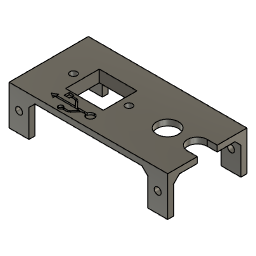
Rear USB Port (Autodesk Fusion 360 design; units mm, degrees)
Autodesk Fusion 360 part; units mm, degrees
note: some values were not read from the file. Set by a fixed rule: which sketch regions a step uses.
sketch "Sketch1" plane through (0, 0, 0) normal (0, 0, 1) x (1, 0, 0)
  line L0 (40, -20) -> (-40, -20)
  line L1 (-40, -20) -> (-40, 20)
  line L2 (-40, 20) -> (40, 20)
  line L3 (40, 20) -> (40, -20)
  line L4 (-20, 5.5) -> (-7, 5.5)
  line L5 (-7, 5.5) -> (-7, -5.5)
  line L6 (-7, -5.5) -> (-20, -5.5)
  line L7 (-20, -5.5) -> (-20, 5.5)
  circle A0 centre (-27.5, 0) radius 1.75
  circle A1 centre (0.5, 0) radius 1.75
  line L8 (-40, -20) -> (-30, -20)
  line L9 (-30, -20) -> (-30, -17)
  line L10 (-30, -17) -> (-40, -17)
  line L11 (-40, -17) -> (-40, -20)
  line L12 (-40, 20) -> (-30, 20)
  line L13 (-30, 20) -> (-30, 17)
  line L14 (-30, 17) -> (-40, 17)
  line L15 (-40, 17) -> (-40, 20)
  line L16 (40, 20) -> (30, 20)
  line L17 (30, 20) -> (30, 17)
  line L18 (30, 17) -> (40, 17)
  line L19 (40, 17) -> (40, 20)
  line L20 (40, -20) -> (30, -20)
  line L21 (30, -20) -> (30, -17)
  line L22 (30, -17) -> (40, -17)
  line L23 (40, -17) -> (40, -20)
  circle A2 centre (20, 0) radius 5.5
  circle A3 centre (35, 0) radius 5
  line L24 (35, 5) -> (35.7366, 5)
  line L25 (35.7366, 5) -> (40, 5)
  line L26 (34.9626, -4.9999) -> (35.7366, -5.0056)
  line L27 (35.7366, -5.0056) -> (40, -5.0056)
  dimension "d1" = 80
  dimension "d2" = 40
  dimension "d3" = 13
  dimension "d4" = 11
  dimension "d5" = 5.5
  dimension "d7" = 3.5
  dimension "d8" = 3.5
  dimension "d9" = 7.5
  dimension "d10" = 7.5
  dimension "d11" = 5.5
  dimension "d12" = 5.5
  dimension "d13" = 10
  dimension "d14" = 3
  dimension "d15" = 3
  dimension "d16" = 10
  dimension "d17" = 3
  dimension "d18" = 10
  dimension "d19" = 10
  dimension "d20" = 3
  dimension "d36" = 14.5
  dimension "d38" = 20
  dimension "d39" = 40
  dimension "d40" = 11
  dimension "d42" = 20
  dimension "d43" = 10
  dimension "d44" = 5
  dimension "d45" = 15
  constraint perpendicular L0 L1
  constraint parallel L0 L2
  constraint parallel L1 L3
  constraint horizontal L0
  constraint horizontal L4
  constraint vertical L5
  constraint horizontal L6
  constraint vertical L7
  constraint horizontal L8
  constraint vertical L9
  constraint horizontal L10
  constraint vertical L11
  constraint horizontal L12
  constraint vertical L13
  constraint horizontal L14
  constraint vertical L15
  constraint horizontal L16
  constraint vertical L17
  constraint horizontal L18
  constraint vertical L19
  constraint horizontal L20
  constraint vertical L21
  constraint horizontal L22
  constraint vertical L23
  constraint coincident A3 L24.start
  constraint tangent A3 L24
  constraint perpendicular L3 L24
  constraint coincident L3 L25.end
  constraint perpendicular L3 L25
  constraint coincident A3 L26.start
  constraint tangent A3 L26
  constraint coincident L3 L27.end
  constraint perpendicular L3 L27
  measures "d1" distance of L1.end L2.end
  measures "d2" distance of L0.end L1.end
  measures "d3" distance of L4.start L4.end
  measures "d4" distance of L4.start L6.end
  measures "d5" distance of origin L4
  measures "d7" diameter of A0
  measures "d8" diameter of A1
  measures "d9" distance of L5 A1.centre
  measures "d10" distance of L7 A0.centre
  measures "d11" distance of L4 A1.centre
  measures "d12" distance of L4 A0.centre
  measures "d13" distance of L0.end L8.end
  measures "d14" distance of L0.end L10.end
  measures "d15" distance of L1.end L14.end
  measures "d16" distance of L1.end L12.end
  measures "d17" distance of L2.end L18.end
  measures "d18" distance of L2.end L16.end
  measures "d19" distance of L0.start L20.end
  measures "d20" distance of L0.start L22.end
  measures "d36" distance of L2 L4
  measures "d38" distance of L1 L7
  measures "d39" distance of L3 origin
  measures "d40" diameter of A2
  measures "d42" distance of L2 A2.centre
  measures "d43" diameter of A3
  measures "d44" distance of L3 A3.centre
  measures "d45" distance of A2.centre A3.centre
extrude "Extrude1" add sketch "Sketch1" along normal blind 3 contours L0 L3 L20 L21 L22 L23 | L0 L1 L2 L3 L9 L10 L13 L14 L17 L18 L21 L22 A3 L24 L25 L26 L27 | L0 L1 L8 L9 L10 L11 | L1 L2 L12 L13 L14 L15 | L2 L3 L16 L17 L18 L19
extrude "Extrude2" add sketch "Sketch1" against normal blind 17 contours L0 L3 L20 L21 L22 L23 | L0 L1 L8 L9 L10 L11 | L1 L2 L12 L13 L14 L15 | L2 L3 L16 L17 L18 L19
sketch "Sketch2" plane through (0, -20, 0) normal (0, -1, 0) x (1, 0, 0)
  line L0 (-30, 0) -> (30, 0)
  line L1 (30, 0) -> (30, -17)
  line L2 (30, -17) -> (40, -17)
  line L3 (40, -17) -> (40, 3)
  line L4 (40, 3) -> (-40, 3)
  line L5 (-40, 3) -> (-40, -17)
  line L6 (-40, -17) -> (-30, -17)
  line L7 (-30, -17) -> (-30, 0)
  circle A0 centre (35, -7) radius 1.75
  circle A1 centre (-35, -7) radius 1.75
  dimension "d25" = 3.5
  dimension "d26" = 10
  dimension "d27" = 5
  dimension "d28" = 3.5
  dimension "d29" = 5
  dimension "d30" = 10
  measures "d25" diameter of A0
  measures "d26" distance of L4 A0.centre
  measures "d27" distance of L3 A0.centre
  measures "d28" diameter of A1
  measures "d29" distance of L5 A1.centre
  measures "d30" distance of L4 A1.centre
extrude "Extrude3" cut sketch "Sketch2" against normal up to surface (40 mm away) contours A0 | A1
chamfer "Chamfer1" distance 3 angle 45 4 edges at (-7, 0, 3) (-13.5, 5.5, 3) (-20, 0, 3) (-13.5, -5.5, 3)
sketch "Sketch3" plane through (0, 0, 3) normal (0, 0, 1) x (-1, 0, 0)
  line L0 (-40, -5) -> (-40, -20)
  line L1 (-40, -20) -> (40, -20)
  line L2 (40, -20) -> (40, 20)
  circle A0 centre (27.5, 0) radius 1.75
  circle A1 centre (-0.5, 0) radius 1.75
  line L3 (23, 8.5) -> (23, -8.5)
  line L4 (23, -8.5) -> (4, -8.5)
  line L5 (4, -8.5) -> (4, 8.5)
  line L6 (4, 8.5) -> (23, 8.5)
  line L7 (24.6533, 14.1697) -> (22.2252, 15.5719)
  line L8 (22.2252, 15.5719) -> (22.2252, 14.5716)
  line L9 (22.2252, 14.5716) -> (9.8144, 14.5716)
  line L10 (9.8144, 14.5716) -> (12.2309, 17.1247)
  spline S0 degree 3 poles (12.2309, 17.1247) (12.4366, 17.2895) (12.7057, 17.4052) (12.9824, 17.4116) knots 0 0 0 0 1 1 1 1
  spline S1 degree 3 poles (12.9824, 17.4116) (14.1022, 17.4116) (14.7671, 17.4119) (15.0119, 17.4123) knots 0 0 0 0 1 1 1 1
  spline S2 degree 3 poles (15.0119, 17.4123) (15.1778, 16.9396) (15.6235, 16.5985) (16.1533, 16.5985) knots 0 0 0 0 1 1 1 1
  spline S3 degree 3 poles (16.1533, 16.5985) (16.8235, 16.5985) (17.3675, 17.1423) (17.3675, 17.8128) knots 0 0 0 0 1 1 1 1
  spline S4 degree 3 poles (17.3675, 17.8128) (17.3675, 18.4836) (16.8236, 19.0273) (16.1533, 19.0273) knots 0 0 0 0 1 1 1 1
  spline S5 degree 3 poles (16.1533, 19.0273) (15.6235, 19.0273) (15.1778, 18.6863) (15.0119, 18.214) knots 0 0 0 0 1 1 1 1
  line L11 (15.0119, 18.214) -> (13.0062, 18.2143)
  spline S6 degree 3 poles (13.0062, 18.2143) (12.4626, 18.2143) (11.893, 17.9161) (11.5305, 17.5665) knots 0 0 0 0 1 1 1 1
  spline S7 degree 3 poles (11.5305, 17.5665) (11.5404, 17.5768) (11.5507, 17.5879) (11.5299, 17.5663) knots 0 0 0 0 1 1 1 1
  spline S8 degree 2 poles (11.5299, 17.5663) (11.5222, 17.5576) (8.9661, 14.8578) knots 0 0 0 1 1 1
  spline S9 degree 3 poles (8.9661, 14.8578) (8.7609, 14.6932) (8.4919, 14.5783) (8.2153, 14.5717) knots 0 0 0 0 1 1 1 1
  line L12 (8.2153, 14.5717) -> (6.8114, 14.5717)
  spline S10 degree 3 poles (6.8114, 14.5717) (6.6253, 15.4992) (5.8062, 16.198) (4.8238, 16.198) knots 0 0 0 0 1 1 1 1
  spline S11 degree 3 poles (4.8238, 16.198) (3.7036, 16.198) (2.7957, 15.29) (2.7957, 14.1702) knots 0 0 0 0 1 1 1 1
  spline S12 degree 3 poles (2.7957, 14.1702) (2.7957, 13.0501) (3.7036, 12.142) (4.8238, 12.142) knots 0 0 0 0 1 1 1 1
  spline S13 degree 3 poles (4.8238, 12.142) (5.8064, 12.142) (6.6255, 12.8414) (6.8116, 13.7697) knots 0 0 0 0 1 1 1 1
  line L13 (6.8116, 13.7697) -> (8.1909, 13.7697)
  spline S14 degree 3 poles (8.1909, 13.7697) (8.1945, 13.7697) (8.198, 13.7695) (8.2016, 13.7697) knots 0 0 0 0 1 1 1 1
  line L14 (8.2016, 13.7697) -> (11.2525, 13.7697)
  spline S15 degree 3 poles (11.2525, 13.7697) (11.5285, 13.7626) (11.7971, 13.6476) (12.0022, 13.4828) knots 0 0 0 0 1 1 1 1
  spline S16 degree 2 poles (12.0022, 13.4828) (14.5578, 10.7832) (14.5657, 10.7744) knots 0 0 0 1 1 1
  spline S17 degree 3 poles (14.5657, 10.7744) (14.5861, 10.7527) (14.576, 10.764) (14.5659, 10.7742) knots 0 0 0 0 1 1 1 1
  spline S18 degree 3 poles (14.5659, 10.7742) (14.9284, 10.4246) (15.4982, 10.1266) (16.0419, 10.1266) knots 0 0 0 0 1 1 1 1
  line L15 (16.0419, 10.1266) -> (17.9748, 10.127)
  line L16 (17.9748, 10.127) -> (17.9748, 9.3129)
  line L17 (17.9748, 9.3129) -> (20.4036, 9.3129)
  line L18 (20.4036, 9.3129) -> (20.4036, 11.7414)
  line L19 (20.4036, 11.7414) -> (17.9748, 11.7414)
  line L20 (17.9748, 11.7414) -> (17.9748, 10.9284)
  spline S19 degree 2 poles (17.9748, 10.9284) (17.4657, 10.9293) (16.0182, 10.9293) knots 0 0 0 1 1 1
  spline S20 degree 3 poles (16.0182, 10.9293) (15.7414, 10.9356) (15.472, 11.0511) (15.2665, 11.216) knots 0 0 0 0 1 1 1 1
  line L21 (15.2665, 11.216) -> (12.8494, 13.7695)
  line L22 (12.8494, 13.7695) -> (22.2252, 13.7695)
  line L23 (22.2252, 13.7695) -> (22.2252, 12.7676)
  line L24 (22.2252, 12.7676) -> (24.6533, 14.1697)
  line L25 (-35, -5) -> (-40, -5)
  line L26 (-40, 20) -> (-40, 5.0056)
  line L27 (-40, 5.0056) -> (-35.7366, 5.0056)
  line L28 (-35.7366, 5.0056) -> (-34.9626, 4.9999)
  arc A2 (-35, -5) -> (-34.9626, 4.9999) centre (-35, 0) ccw
  circle A3 centre (-20, 0) radius 5.5
extrude "Extrude4" cut sketch "Sketch3" against normal blind 1 contours L7 L8 L9 L10 S0 S1 S2 S3 S4 S5 L11 S6 S8 S9 L12 S10 S11 S12 S13 L13 S14 L14 S15 S16 S18 L15 L16 L17 L18 L19 L20 S19 S20 L21 L22 L23 L24
extrude "Extrude5" cut sketch "Sketch1" along normal up to surface (3 mm away) contours A3 | A2
chamfer "Chamfer2" distance 3 angle 45 4 edges at (-35, -17, 0) (35, -17, 0) (35, 17, 0) (-35, 17, 0)
chamfer "Chamfer3" distance 3 angle 45 4 edges at (-30, -17, 0) (-30, 17, 0) (30, -17, 0) (30, 17, 0)
equation "d5 = d4 / 2"
equation "d11 = d5"
equation "d12 = d5"
